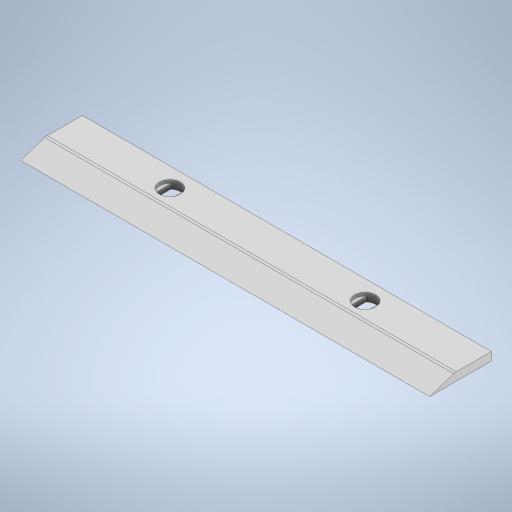
# Autodesk Inventor part: Bladev2
Saved by Autodesk Inventor 2024 (Build 280153000, 153)
## iProperties
Created: 2024-03-09
Part Number: Bladev2
Material: Generic
Document SubType Name: Modeling
Designer: kdcao
Density: 1 g/cm^3
Appearance: Default
Author: kdcao
Autodesk Inventor part; units mm, degrees
ref_plane "YZ Plane" through (0, 0, 0) normal (1, 0, 0) x (0, 1, 0)
ref_plane "XZ Plane" through (0, 0, 0) normal (0, 1, 0) x (-1, 0, 0)
ref_plane "XY Plane" through (0, 0, 0) normal (0, 0, 1) x (1, 0, 0)
sketch "Sketch1" plane through (0, 0, 0) normal (0, 1, 0) x (-1, 0, 0)
  line L0 (-49.75, 7.5) -> (49.75, 7.5)
  line L1 (49.75, 7.5) -> (49.75, -7.5)
  line L2 (49.75, -7.5) -> (-49.75, -7.5)
  line L3 (-49.75, -7.5) -> (-49.75, 7.5)
  line L4 (-49.75, 7.5) -> (49.75, -7.5) construction
  line L5 (49.75, 7.5) -> (-49.75, -7.5) construction
  point P0 (0, 0)
  dimension "d0" = 15
  dimension "d1" = 99.5
  constraints: 12 end point, 2 midpoint, 2 parallel, 1 horizontal, 1 perpendicular
  measures "d0" distance of L0.end L1.end
  measures "d1" distance of L1.end L2.end
extrude "Extrusion1" add sketch "Sketch1" along normal blind 2
sketch "Sketch2" plane through (0, 2, 0) normal (0, 1, 0) x (1, 0, 0)
  line L0 (49.75, 7.5) -> (-49.75, 7.5) projected
  line L1 (49.75, -7.5) -> (49.75, 7.5) projected
  point P0 (0, 0)
  point P1 (23.75, 2.8)
  dimension "d11" = 4.7
  dimension "d12" = 26
  measures "d11" distance from line of L0 point (23.75, 2.8)
  measures "d12" distance from line of L1 point (23.75, 2.8)
hole "Hole1" at (23.75, 2, -2.8) direction (0, -1, 0) diameter 5.1 end through all
sketch "Sketch3" plane through (0, 0, 0) normal (0, -1, 0) x (1, 0, 0)
  line L0 (26.3, -0.25) -> (21.2, -0.25)
  line L1 (21.2, -0.25) -> (21.2, -5.35)
  line L2 (21.2, -5.35) -> (26.3, -5.35)
  line L3 (26.3, -5.35) -> (26.3, -0.25)
  circle A0 centre (23.75, -2.8) radius 2.55 projected
  line L4 (26.3, -0.25) -> (21.2, -5.35) construction
  line L5 (21.2, -0.25) -> (26.3, -5.35) construction
  line L6 (25.3, -5.35) -> (25.3, -0.25)
  line L7 (22.2, -5.35) -> (22.2, -0.25)
  point P0 (0, 0)
  point P1 (22.2, -4.8248)
  point P2 (22.2, -0.7752)
  point P3 (25.3, -0.7752)
  point P4 (25.3, -4.8248)
  dimension "d13" = 5.1
  dimension "d14" = 5.1
  dimension "d15" = 1
  dimension "d16" = 1
  constraints: 16 end point, 4 point on line, 3 perpendicular, 2 midpoint, 2 parallel, 1 horizontal
  measures "d13" distance of L1.end L2.end
  measures "d14" distance of L2.end L0.start
  measures "d15" distance between parallel lines of L3 L6
  measures "d16" distance edge to line of A0 L7
extrude "Extrusion2" add sketch "Sketch3" against normal blind 1.25 contours A0 L6 | L7 A0
fillet "Fillet1" radius 0.2 2 edges at (25.3, 0, -2.8) (22.2, 0, -2.8)
ref_plane "Work Plane1" through (0, 0, -7.5) normal (-1, 0, 0) x (0, 0, 1)
mirror "Mirror1" about plane through (0, 0, -7.5) normal (-1, 0, 0) of "Hole1", "Extrusion2", "Fillet1"
sketch "Sketch4" plane through (-49.75, 0, -7.5) normal (-1, 0, 0) x (0, 0, 1)
  line L0 (0, 0) -> (15, 0) projected
  line L1 (15, 0) -> (8.8446, 2)
  line L2 (0, 2) -> (15, 2) projected
  line L3 (8.8446, 0) -> (15, 0)
  line L4 (8.8446, 2) -> (8.8446, 0)
  line L5 (15, 0) -> (15, 2) projected
  line L6 (8.8446, 2) -> (15, 2)
  line L7 (15, 2) -> (15, 0)
  point P0 (7.5, 0)
  dimension "d21" = 18
  constraints: 10 end point, 1 collinear, 1 horizontal, 1 perpendicular, 1 point on line, 1 vertical
  measures "d21" angle of L0 L1
extrude "Extrusion3" cut sketch "Sketch4" against normal through all contours L1 L2 L5
fillet "Fillet2" radius 2 1 edges at (0, 2, 1.3446)
body "Solid1"
